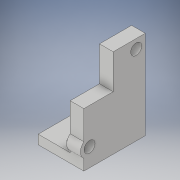
# Autodesk Inventor part: Ultrasonic MoUnt
Saved by Autodesk Inventor 2018 (Build 220112000, 112)
## iProperties
Created: 2018-02-23
Part Number: Ultrasonic MoUnt
Material: Generic
Document SubType Name: Modeling
Designer: MIABo
Density: 1 g/cm^3
Appearance: Default
Mass: 1.62456 g
Surface Area: 14.2231 cm^2
Volume: 1.62456 cm^3
Author: MIABo
Autodesk Inventor part; units mm, degrees
ref_plane "YZ Plane" through (0, 0, 0) normal (1, 0, 0) x (0, 1, 0)
ref_plane "XZ Plane" through (0, 0, 0) normal (0, 1, 0) x (-1, 0, 0)
ref_plane "XY Plane" through (0, 0, 0) normal (0, 0, 1) x (1, 0, 0)
sketch "Sketch1" plane through (0, 0, 0) normal (0, 1, 0) x (-1, 0, 0)
  line L0 (20.8788, 34.798) -> (8.1788, 34.798)
  line L1 (8.1788, 34.798) -> (8.1788, 17.7292)
  line L2 (8.1788, 17.7292) -> (20.8788, 17.7292)
  line L3 (20.8788, 17.7292) -> (20.8788, 34.798)
  point P0 (0, 0)
  dimension "d0" = 17.0688
  dimension "d1" = 12.7
  constraints: 8 end point, 2 parallel, 1 horizontal, 1 perpendicular
  measures "d0" distance of L2.end L0.start
  measures "d1" distance of L0.start L0.end
extrude "Extrusion1" add sketch "Sketch1" along normal blind 2.54
sketch "Sketch2" plane through (0, 2.54, 0) normal (0, 1, 0) x (1, 0, 0)
  line L0 (-8.1788, -17.7292) -> (-20.8788, -17.7292) projected
  line L1 (-20.8788, -34.798) -> (-8.1788, -34.798) projected
  line L2 (-20.8788, -17.7292) -> (-20.8788, -34.798) projected
  point P0 (0, 0)
  point P1 (-14.5288, -31.623)
  point P2 (-14.5288, -20.9042)
  dimension "d5" = 3.175
  dimension "d6" = 3.175
  dimension "d14" = 6.35
  dimension "d15" = 6.35
  measures "d5" distance from line of L1 point (-14.529, -31.623)
  measures "d6" distance from line of L0 point (-14.529, -20.904)
  measures "d14" distance from line of L2 point (-14.529, -31.623)
  measures "d15" distance from line of L2 point (-14.529, -20.904)
hole "Hole1" at (-14.5288, 2.54, 31.623) at (-14.5288, 2.54, 20.9042) direction (0, -1, 0) diameter 2.2098 end through all
sketch "Sketch4" plane through (0, 2.54, 0) normal (0, 1, 0) x (1, 0, 0)
  line L0 (-8.1788, -34.798) -> (-8.1788, -17.7292) projected
  line L1 (-20.8788, -34.798) -> (-8.1788, -34.798) projected
  line L2 (-8.1788, -17.7292) -> (-11.9888, -17.7292)
  line L3 (-11.9888, -17.7292) -> (-11.9888, -34.798)
  line L4 (-11.9888, -34.798) -> (-8.1788, -34.798)
  line L5 (-8.1788, -34.798) -> (-8.1788, -17.7292)
  point P0 (0, 0)
  dimension "d16" = 3.81
  constraints: 8 end point, 2 parallel, 1 horizontal, 1 perpendicular, 1 point on line
  measures "d16" distance of L0.end L2.end
extrude "Extrusion2" add sketch "Sketch4" along normal blind 22.098
sketch "Sketch5" plane through (-8.1788, 0, 34.798) normal (1, 0, 0) x (0, 0, -1)
  line L0 (0, 24.638) -> (17.0688, 24.638) projected
  line L1 (0, 0) -> (0, 24.638) projected
  line L2 (17.0688, 0) -> (17.0688, 24.638) projected
  point P0 (34.798, 0)
  point P1 (1.5748, 5.08)
  point P2 (14.5288, 22.098)
  dimension "d26" = 2.54
  dimension "d27" = 2.54
  dimension "d29" = 17.018
  dimension "d31" = 15.494
  measures "d26" distance from line of L0 point (14.529, 22.098)
  measures "d27" distance from line of L2 point (14.529, 22.098)
  measures "d29" vertical distance of point (1.575, 5.08) point (14.529, 22.098)
  measures "d31" distance from line of L2 point (1.575, 5.08)
hole "Hole2" at (-8.1788, 5.08, 33.2232) at (-8.1788, 22.098, 20.2692) direction (-1, 0, 0) diameter 3.048 end through all
sketch "Sketch6" plane through (-8.1788, 0, 34.798) normal (1, 0, 0) x (0, 0, -1)
  circle A0 centre (1.5748, 5.08) radius 2.54
  circle A1 centre (1.5748, 5.08) radius 1.524 projected
  point P0 (34.798, 0)
  dimension "d51" = 5.08
  constraints: 1 centre point, 1 concentric
  measures "d51" diameter of A0
extrude "Extrusion3" add sketch "Sketch6" against normal up to surface (3.81 mm away)
sketch "Sketch7" plane through (-8.1788, 0, 34.798) normal (1, 0, 0) x (0, 0, -1)
  line L0 (0, 24.638) -> (17.0688, 24.638) projected
  line L1 (0, 24.638) -> (8.1534, 24.638)
  line L2 (8.1534, 24.638) -> (8.1534, 15.0368)
  line L3 (8.1534, 15.0368) -> (0, 15.0368)
  line L4 (0, 15.0368) -> (0, 24.638)
  line L5 (17.0688, 0) -> (17.0688, 24.638) projected
  line L6 (0, 7.0729) -> (0, 24.638) projected
  dimension "d44" = 9.6012
  dimension "d46" = 8.9154
  constraints: 8 end point, 2 parallel, 1 collinear, 1 horizontal, 1 perpendicular, 1 point on line
  measures "d44" distance of L3.end L1.start
  measures "d46" distance between parallel lines of L5 L2
extrude "Extrusion4" cut sketch "Sketch7" against normal blind 22.098
body "Solid1"
